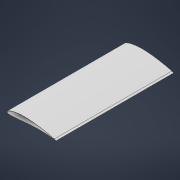
# Autodesk Inventor part: wing
Saved by Autodesk Inventor 2022 (Build 260153000, 153)
## iProperties
Created: 2022-11-19
Part Number: wing
Material: Generic
Document SubType Name: Modeling
Designer: Maciej
Density: 1 g/cm^3
Appearance: Default
Author: Maciej
Autodesk Inventor part; units mm, degrees
ref_plane "YZ Plane" through (0, 0, 0) normal (1, 0, 0) x (0, 1, 0)
ref_plane "XZ Plane" through (0, 0, 0) normal (0, 1, 0) x (-1, 0, 0)
ref_plane "XY Plane" through (0, 0, 0) normal (0, 0, 1) x (1, 0, 0)
sketch "Sketch1" plane through (0, 0, 0) normal (0, 0, 1) x (1, 0, 0)
  spline S0 degree 5 poles (200, 0) (200.0794, 0.3654) (193.4187, 2.2512) (166.3713, 8.3099) (164.9342, 8.4484) (136.8126, 13.7759) (121.4131, 15.9413) (99.1179, 18.1167) (81.6456, 19.3989) (59.1788, 18.5848) (47.9019, 17.966) (22.1067, 13.8656) (16.4956, 10.9775) (12.1395, 9.9238) (4.0847, 5.4489) (4.0794, 5.1268) (-3.1285, -0.125) (3.7014, -3.4576) (4.2933, -3.5118) (12.321, -4.6307) (16.6127, -4.7711) (22.5637, -4.3012) (48.2671, -3.0804) (59.2014, -1.144) (81.6846, 0.4504) (98.9987, 2.5809) (121.3043, 2.6002) (136.7028, 4.5049) (164.7468, 1.7799) (166.5085, 4.3351) (193.1478, 0.2865) (199.9216, -0.3612) (200, 0) knots 0 0 0 0 0 0 0.053298 0.088722 0.132936 0.177011 0.220992 0.264924 0.308901 0.348598 0.384091 0.415494 0.44157 0.463031 0.483758 0.503099 0.522165 0.54216 0.562296 0.587432 0.618172 0.653295 0.69281 0.736712 0.780608 0.824485 0.868348 0.912219 0.947318 1 1 1 1 1 1
  spline S1 degree 4 poles (200.2516, 0.9678) (187.839, 4.6756) (170.3627, 8.5167) (147.7708, 12.9791) (120.2421, 17.1037) (99.9728, 19.0359) (80.4054, 20.3107) (59.4226, 19.5973) (44.6969, 18.6661) (20.9909, 14.1992) (15.9627, 12.0469) (10.3137, 10.0603) (3.9964, 6.4499) (2.401, 5.4049) (-3.2597, -0.1511) (2.4015, -4.1671) (4.4188, -4.5464) (10.7646, -5.4149) (16.3885, -5.8201) (21.5277, -5.3313) (45.1882, -4.2281) (59.6054, -2.2736) (80.4804, -0.5) (99.882, 1.3589) (120.0765, 1.9403) (147.4508, 3.1981) (170.0113, 1.2714) (187.4322, 1.0042) (199.9005, -0.995) knots 0 0 0 0 0 0.110201 0.154058 0.19781 0.241488 0.28515 0.328916 0.367426 0.400748 0.429003 0.4507 0.472444 0.493673 0.513237 0.533866 0.554292 0.574996 0.602398 0.635179 0.673373 0.71698 0.760566 0.804116 0.847634 0.891138 1 1 1 1 1
  line L0 (199.9005, -0.995) -> (208, -2)
  line L1 (200.2516, 0.9678) -> (208, -2)
  point P0 (160, 9.4)
  point P1 (140, 13)
  point P2 (120, 15.9)
  point P3 (100, 17.9)
  point P4 (80, 18.9)
  point P5 (60, 18.5)
  point P6 (40, 16.5)
  point P7 (20, 12.4)
  point P8 (15, 10.676)
  point P9 (10, 8.55)
  point P10 (5, 5.824)
  point P11 (2.5, 3.962)
  point P12 (0, 0)
  point P13 (2.5, -2.738)
  point P14 (5, -3.576)
  point P15 (10, -4.25)
  point P16 (15, -4.626)
  point P17 (20, -4.5)
  point P18 (40, -3.3)
  point P19 (60, -1.4)
  point P20 (80, 0.5)
  point P21 (100, 2.1)
  point P22 (120, 3)
  point P23 (140, 3.5)
  point P24 (160, 3)
  point P25 (180, 2)
  point P26 (180.2286, 6.1735)
  point P27 (160.1914, 10.3815)
  point P28 (140.1603, 13.9871)
  point P29 (120.1215, 16.8926)
  point P30 (100.0747, 18.8972)
  point P31 (80.015, 19.8999)
  point P32 (59.9402, 19.4982)
  point P33 (39.8496, 17.4886)
  point P34 (19.736, 13.3645)
  point P35 (14.6411, 11.6094)
  point P36 (9.5645, 9.4502)
  point P37 (4.4607, 6.6661)
  point P38 (1.7661, 4.6413)
  point P39 (-0.9961, -0.0884)
  point P40 (1.9544, -3.576)
  point P41 (4.7733, -4.55)
  point P42 (9.8957, -5.2445)
  point P43 (14.9751, -5.6257)
  point P44 (20.0425, -5.4991)
  point P45 (40.0772, -4.297)
  point P46 (60.0946, -2.3955)
  point P47 (80.0872, -0.4962)
  point P48 (100.0624, 1.1019)
  point P49 (120.035, 2.0006)
  point P50 (140, 2.5)
  point P51 (159.9625, 2.0007)
  point P52 (179.9253, 1.0028)
  constraints: 4 end point, 57 other
sketch "Sketch2" plane through (0, 0, 0) normal (0, 0, 1) x (1, 0, 0)
  point P0 (0, 0)
extrude "Extrusion1" add sketch "Sketch1" along normal mid plane 500
body "Solid1"
